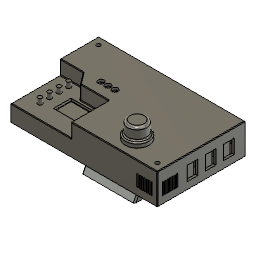
Cover Control Gehäuse (Autodesk Fusion 360 design; units mm, degrees)
Autodesk Fusion 360 part; units mm, degrees
sketch "Skizze1" plane through (0, 0, 0) normal (0, 1, 0) x (1, 0, 0)
  line L0 (0, 0) -> (120, 0)
  line L1 (120, 0) -> (120, -70)
  line L2 (120, -70) -> (0, -70)
  line L3 (0, -70) -> (0, 0)
  circle A0 centre (4, -4) radius 1.6
  circle A1 centre (4, -66) radius 1.6
  circle A2 centre (116, -66) radius 1.6
  circle A3 centre (64, -4) radius 1.6
  dimension "d1" = 120
  dimension "d2" = 70
  dimension "d3" = 3.2
  dimension "d4" = 3.2
  dimension "d5" = 3.2
  dimension "d7" = 3.2
  constraint horizontal L0
  constraint vertical L1
  constraint horizontal L2
  constraint vertical L3
  constraint coincident L0.start L3.end
  measures "d1" distance of L0.start L0.end
  measures "d2" distance of L0.start L2.end
  measures "d3" diameter of A0
  measures "d4" diameter of A1
  measures "d5" diameter of A2
  measures "d7" diameter of A3
extrude "Extrusion1" add sketch "Skizze1" along normal blind 1.6 makes body 1
sketch "Skizze2" plane through (0, 1.6, 0) normal (0, 1, 0) x (-1, 0, 0)
  circle A0 centre (-4, 66) radius 1.6
  circle A1 centre (-64, 4) radius 1.6
  circle A2 centre (-116, 66) radius 1.6
  circle A3 centre (-4, 4) radius 1.6
  line L0 (0, 70) -> (-120, 70)
  line L1 (-120, 70) -> (-120, 0)
  line L2 (-120, 0) -> (0, 0)
  line L3 (0, 0) -> (0, 70)
  line L4 (0, 70) -> (-10, 70)
  line L5 (-10, 70) -> (-10, 60)
  line L6 (-10, 60) -> (0, 60)
  line L7 (0, 60) -> (0, 70)
  line L8 (-10, 60) -> (-10, 51.86)
  line L9 (-10, 51.86) -> (-10, 43.72)
  line L10 (-10, 43.72) -> (-10, 35.58)
  circle A4 centre (-10, 60) radius 1.75
  circle A5 centre (-10, 35.58) radius 1.75
  circle A6 centre (-10, 51.86) radius 1.75
  circle A7 centre (-10, 43.72) radius 1.75
  line L11 (0, 70) -> (-19.44, 70)
  line L12 (-19.44, 70) -> (-19.44, 58)
  line L13 (-19.44, 58) -> (0, 58)
  line L14 (0, 58) -> (0, 70)
  line L15 (-19.44, 58) -> (-46.94, 58)
  line L16 (-46.94, 58) -> (-46.94, 43)
  line L17 (-46.94, 43) -> (-19.44, 43)
  line L18 (-19.44, 43) -> (-19.44, 58)
  line L19 (-120, 70) -> (-94, 70)
  line L20 (-94, 70) -> (-94, 61.2)
  line L21 (-94, 61.2) -> (-120, 61.2)
  line L22 (-120, 61.2) -> (-120, 70)
  circle A8 centre (-94, 61.2) radius 3.5
  line L23 (0, 70) -> (0, 30)
  line L24 (0, 30) -> (-32, 30)
  circle A9 centre (-32, 30) radius 2.4
  line L25 (-32, 30) -> (-38, 30)
  circle A10 centre (-38, 30) radius 2.4
  line L26 (-38, 30) -> (-44, 30)
  circle A11 centre (-44, 30) radius 2.4
  line L27 (0, 0) -> (-16, 0)
  line L28 (-16, 0) -> (-25, 0)
  line L29 (-25, 0) -> (-25, 14)
  line L30 (-25, 14) -> (-16, 14)
  line L31 (-16, 14) -> (-16, 0)
  line L32 (0, 0) -> (-66, 0)
  line L33 (-120, 8) -> (-106, 8)
  line L34 (-106, 8) -> (-106, 17)
  line L35 (-106, 17) -> (-120, 17)
  line L36 (-120, 17) -> (-120, 8)
  line L37 (-120, 17) -> (-120, 23.5)
  line L38 (-120, 23.5) -> (-106, 23.5)
  line L39 (-106, 23.5) -> (-106, 32.5)
  line L40 (-106, 32.5) -> (-120, 32.5)
  line L41 (-120, 32.5) -> (-120, 23.5)
  line L42 (-120, 32.5) -> (-120, 39)
  line L43 (-120, 39) -> (-106, 39)
  line L44 (-106, 39) -> (-106, 48)
  line L45 (-106, 48) -> (-120, 48)
  line L46 (-120, 48) -> (-120, 39)
  line L47 (-120, 70) -> (-118, 70)
  line L48 (-118, 70) -> (-118, 64)
  line L49 (-118, 64) -> (-120, 64)
  line L50 (-120, 64) -> (-120, 70)
  line L51 (-118, 64) -> (-104, 64)
  line L52 (-104, 64) -> (-104, 54)
  line L53 (-104, 54) -> (-118, 54)
  line L54 (-118, 54) -> (-118, 64)
  line L55 (-66, 0) -> (-76, 0)
  line L56 (-76, 0) -> (-76, 10)
  line L57 (-76, 10) -> (-66, 10)
  line L58 (-66, 10) -> (-66, 0)
  line L59 (-120, 0) -> (-76, 0)
  line L60 (-76, 0) -> (-51, 0)
  line L61 (-51, 0) -> (-51, 66)
  line L62 (-51, 66) -> (-76, 66)
  line L63 (-76, 66) -> (-76, 0)
  line L64 (-66, 0) -> (-56, 0)
  line L65 (-56, 0) -> (-56, 10)
  line L66 (-56, 10) -> (-66, 10)
  line L67 (-66, 10) -> (-66, 0)
  dimension "d10" = 10
  dimension "d11" = 10
  dimension "d12" = 8.14
  dimension "d13" = 8.14
  dimension "d14" = 8.14
  dimension "d15" = 3.5
  dimension "d17" = 3.5
  dimension "d18" = 3.5
  dimension "d19" = 3.5
  dimension "d20" = 19.44
  dimension "d21" = 12
  dimension "d22" = 27.5
  dimension "d23" = 15
  dimension "d24" = 26
  dimension "d25" = 8.8
  dimension "d26" = 7
  dimension "d27" = 40
  dimension "d28" = 32
  dimension "d29" = 4.8
  dimension "d30" = 6
  dimension "d31" = 4.8
  dimension "d32" = 6
  dimension "d33" = 4.8
  dimension "d34" = 16
  dimension "d35" = 9
  dimension "d36" = 14
  dimension "d37" = 66
  dimension "d38" = 14
  dimension "d39" = 9
  dimension "d40" = 6.5
  dimension "d41" = 14
  dimension "d42" = 9
  dimension "d43" = 6.5
  dimension "d44" = 14
  dimension "d45" = 9
  dimension "d46" = 2
  dimension "d47" = 6
  dimension "d48" = 14
  dimension "d49" = 10
  dimension "d62" = 10
  dimension "d63" = 10
  dimension "d64" = 44
  dimension "d65" = 25
  dimension "d66" = 66
  dimension "d67" = 10
  dimension "d68" = 10
  constraint horizontal L4
  constraint vertical L5
  constraint horizontal L6
  constraint vertical L7
  constraint coincident L0.start L3.end
  constraint perpendicular L6 L8
  constraint parallel L8 L9
  constraint parallel L9 L10
  constraint coincident L5.end L6.start
  constraint coincident L10.end A5.centre
  constraint coincident L8.end L9.start
  constraint coincident L9.end L10.start
  constraint horizontal L11
  constraint vertical L12
  constraint horizontal L13
  constraint vertical L14
  constraint horizontal L15
  constraint vertical L16
  constraint horizontal L17
  constraint vertical L18
  constraint horizontal L19
  constraint vertical L20
  constraint horizontal L21
  constraint vertical L22
  constraint coincident L0.end L1.start
  constraint coincident L20.end L21.start
  constraint perpendicular L4 L23
  constraint perpendicular L23 L24
  constraint coincident L24.end A9.centre
  constraint parallel L24 L25
  constraint coincident L25.end A10.centre
  constraint parallel L25 L26
  constraint coincident L26.end A11.centre
  constraint coincident L2.end L3.start
  constraint perpendicular L3 L27
  constraint horizontal L28
  constraint vertical L29
  constraint horizontal L30
  constraint vertical L31
  constraint parallel L2 L32
  constraint horizontal L33
  constraint vertical L34
  constraint horizontal L35
  constraint vertical L36
  constraint coincident L1 L33.start
  constraint perpendicular L35 L37
  constraint horizontal L38
  constraint vertical L39
  constraint horizontal L40
  constraint vertical L41
  constraint perpendicular L40 L42
  constraint horizontal L43
  constraint vertical L44
  constraint horizontal L45
  constraint vertical L46
  constraint horizontal L47
  constraint vertical L48
  constraint horizontal L49
  constraint vertical L50
  constraint horizontal L51
  constraint vertical L52
  constraint horizontal L53
  constraint vertical L54
  constraint horizontal L55
  constraint vertical L56
  constraint horizontal L57
  constraint vertical L58
  constraint coincident L1.end L2.start
  constraint perpendicular L1 L59
  constraint horizontal L60
  constraint vertical L61
  constraint horizontal L62
  constraint vertical L63
  constraint horizontal L64
  constraint vertical L65
  constraint horizontal L66
  constraint vertical L67
  measures "d5" diameter of L10.end
  measures "d10" distance of L0.start L4.end
  measures "d11" distance of L0.start L6.end
  measures "d12" distance of L5.end L8.end
  measures "d13" distance of L8.end L9.end
  measures "d14" distance of L9.end L10.end
  measures "d15" diameter of A4
  measures "d17" diameter of A5
  measures "d18" diameter of A6
  measures "d19" diameter of A7
  measures "d20" distance of L0.start L11.end
  measures "d21" distance of L0.start L13.end
  measures "d22" distance of L12.end L15.end
  measures "d23" distance of L12.end L17.end
  measures "d24" distance of L0.end L19.end
  measures "d25" distance of L0.end L21.end
  measures "d26" diameter of A8
  measures "d27" distance of L0.start L23.end
  measures "d28" distance of L23.end L24.end
  measures "d29" diameter of A9
  measures "d30" distance of L24.end L25.end
  measures "d31" diameter of A10
  measures "d32" distance of L25.end L26.end
  measures "d33" diameter of A11
  measures "d34" distance of L2.end L27.end
  measures "d35" distance of L27.end L28.end
  measures "d36" distance of L27.end L30.end
  measures "d37" distance of L2.end L32.end
  measures "d38" distance of L33.start L33.end
  measures "d39" distance of L33.start L35.end
  measures "d40" distance of L35.end L37.end
  measures "d41" distance of L37.end L38.end
  measures "d42" distance of L37.end L40.end
  measures "d43" distance of L40.end L42.end
  measures "d44" distance of L42.end L43.end
  measures "d45" distance of L42.end L45.end
  measures "d46" distance of L0.end L47.end
  measures "d47" distance of L0.end L49.end
  measures "d48" distance of L48.end L51.end
  measures "d49" distance of L48.end L53.end
  measures "d62" distance of L32.end L55.end
  measures "d63" distance of L32.end L57.end
  measures "d64" distance of L1.end L55.end
  measures "d65" distance of L55.end L60.end
  measures "d66" distance of L55.end L62.end
  measures "d67" distance of L32.end L64.end
  measures "d68" distance of L32.end L57.end
  measures "d89" diameter of L35.end
  measures "d93" diameter of L10.end
  measures "d96" diameter of L35.end
extrude "Extrusion2" add sketch "Skizze2" along normal blind 11 contours L2 L28 L29 L30 L31 L32 | L1 L43 L44 L45 L46 | L1 L38 L39 L40 L41 | L1 L33 L34 L35 L36 bodies 1
extrude "Extrusion3" add sketch "Skizze2" along normal blind 5 contours L21 L51 L52 L54 | L21 L52 L53 L54 bodies 1
extrude "Extrusion4" add sketch "Skizze2" along normal blind 6 contours L15 L16 L17 L18 bodies 1
extrude "Extrusion5" add sketch "Skizze2" along normal blind 13 contours L5 L6 A4 | L5 L8 A4 | L6 L8 A4 | L8 L9 A6 | L8 L9 A6 | L9 L10 A7 | L9 L10 A7 | A5 bodies 1
extrude "Extrusion6" add sketch "Skizze2" along normal blind 12.5 contours L24 A9 L25 | L24 A9 L25 | L25 A10 L26 | L25 A10 L26 | A11 bodies 1
extrude "Extrusion7" add sketch "Skizze2" along normal blind 25 contours L20 L21 A8 | L20 L21 A8 bodies 1
extrude "Extrusion8" add sketch "Skizze2" along normal blind 10.3 contours L2 L55 L56 L57 L58 L60 L63 L67 bodies 1
extrude "Extrusion9" add sketch "Skizze2" along normal blind 12.3 contours L2 L32 L58 L60 L64 L65 L66 L67 bodies 1
extrude "Extrusion10" add sketch "Skizze2" along normal blind 9.5 contours L2 L32 L57 L60 L61 L62 L63 L65 L66 bodies 1
sketch "Skizze3" plane through (0, 0, 0) normal (0, 1, 0) x (1, 0, 0)
  line L0 (120, -70) -> (122.5, -70)
  line L1 (122.5, -70) -> (122.5, -72.5)
  line L2 (122.5, -72.5) -> (120, -72.5)
  line L3 (120, -72.5) -> (120, -70)
  line L4 (0, 0) -> (-2.5, 0)
  line L5 (-2.5, 0) -> (-2.5, 2.5)
  line L6 (-2.5, 2.5) -> (0, 2.5)
  line L7 (0, 2.5) -> (0, 0)
  line L8 (-2.5, 2.5) -> (122.5, 2.5)
  line L9 (122.5, 2.5) -> (122.5, -72.5)
  line L10 (122.5, -72.5) -> (-2.5, -72.5)
  line L11 (-2.5, -72.5) -> (-2.5, 2.5)
  dimension "d75" = 2.5
  dimension "d76" = 2.5
  dimension "d77" = 2.5
  dimension "d78" = 2.5
  constraint horizontal L0
  constraint vertical L1
  constraint horizontal L2
  constraint vertical L3
  constraint horizontal L4
  constraint vertical L5
  constraint horizontal L6
  constraint vertical L7
  constraint coincident L4.start L7.end
  constraint horizontal L8
  constraint vertical L9
  constraint horizontal L10
  constraint vertical L11
  measures "d75" distance of L0.start L0.end
  measures "d76" distance of L0.start L2.end
  measures "d77" distance of L4.start L4.end
  measures "d78" distance of L4.start L6.end
extrude "Extrusion11" add sketch "Skizze3" along normal blind 22 separate body makes body 2
sketch "Skizze4" plane through (0, 22, 0) normal (0, 1, 0) x (-1, 0, 0)
  line L0 (2.5, 72.5) -> (-122.5, 72.5)
  line L1 (-122.5, 72.5) -> (-122.5, -2.5)
  line L2 (-122.5, -2.5) -> (2.5, -2.5)
  line L3 (2.5, -2.5) -> (2.5, 72.5)
  line L4 (2.5, 72.5) -> (-49, 72.5)
  line L5 (-49, 72.5) -> (-49, 40.5)
  line L6 (-49, 40.5) -> (-25, 40.5)
  line L7 (-25, 40.5) -> (-17.4344, 30.5702)
  line L8 (-17.4344, 30.5702) -> (2.5, 30.5702)
  dimension "d81" = 51.5
  dimension "d82" = 32
  dimension "d83" = 24
  constraint coincident L0.start L3.end
  constraint perpendicular L3 L4
  constraint perpendicular L4 L5
  constraint perpendicular L5 L6
  constraint coincident L3 L8.end
  constraint perpendicular L3 L8
  measures "d81" distance of L0.start L4.end
  measures "d82" distance of L4.end L5.end
  measures "d83" distance of L5.end L6.end
extrude "Extrusion12" cut sketch "Skizze4" against normal blind 12 contours L0 L3 L4 L5 L6 L7 L8 bodies 2
shell "Schale1" thickness 2 removed faces 1 at (80.8333, 0, 47.5) on bodies 2
sketch "Skizze6" plane through (0, 20, 0) normal (0, -1, 0) x (1, 0, 0)
  line L0 (51, 70.5) -> (51, 38.5)
  line L1 (51, 38.5) -> (25.9905, 38.5)
  line L2 (25.9905, 38.5) -> (18.425, 28.5702)
  line L3 (18.425, 28.5702) -> (-0.5, 28.5702)
  line L4 (-0.5, 28.5702) -> (-0.5, -0.5)
  line L5 (-0.5, -0.5) -> (120.5, -0.5)
  line L6 (120.5, -0.5) -> (120.5, 70.5)
  line L7 (120.5, 70.5) -> (51, 70.5)
  line L8 (120.5, 70.5) -> (102.5114, 70.5)
  line L9 (102.5114, 70.5) -> (102.5114, 51.9822)
  line L10 (102.5114, 51.9822) -> (120.5, 51.9822)
  line L11 (120.5, 51.9822) -> (120.5, 70.5)
  line L12 (120.5, 70.5) -> (101.404, 70.5)
  line L13 (101.404, 70.5) -> (101.404, 51.0001)
  line L14 (101.404, 51.0001) -> (120.5, 51.0001)
  line L15 (120.5, 51.0001) -> (120.5, 70.5)
  constraint horizontal L8
  constraint vertical L9
  constraint horizontal L10
  constraint vertical L11
  constraint coincident L6.end L7.start
  constraint horizontal L12
  constraint vertical L13
  constraint horizontal L14
  constraint vertical L15
extrude "Extrusion13" add sketch "Skizze6" along normal blind 18 contours L6 L7 L9 L10 L12 L13 L14 L15 bodies 2
sketch "Skizze7" plane through (0, 10, 0) normal (0, 1, 0) x (-1, 0, 0)
  line L0 (-17.4344, 30.5702) -> (2.5, 30.5702)
  line L1 (2.5, 30.5702) -> (2.5, 72.5)
  line L2 (2.5, 72.5) -> (-49, 72.5)
  line L3 (-49, 72.5) -> (-49, 40.5)
  line L4 (-49, 40.5) -> (-25, 40.5)
  line L5 (-25, 40.5) -> (-17.4344, 30.5702)
  line L6 (-19.5, 42.9671) -> (-47, 42.9671)
  line L7 (-47, 42.9671) -> (-47, 57.9671)
  line L8 (-47, 57.9671) -> (-19.5, 57.9671)
  line L9 (-19.5, 57.9671) -> (-19.5, 42.9671)
  circle A0 centre (-10, 60) radius 1.9
  circle A1 centre (-10, 35.6) radius 1.9
  circle A2 centre (-9.9957, 43.7481) radius 1.9
  circle A3 centre (-10, 51.85) radius 1.9
  dimension "d89" = 3.8
  dimension "d91" = 3.8
  dimension "d92" = 3.8
  dimension "d93" = 3.8
  constraint horizontal L6
  constraint vertical L7
  constraint horizontal L8
  constraint vertical L9
  measures "d89" diameter of A0
  measures "d91" diameter of A1
  measures "d92" diameter of A2
  measures "d93" diameter of A3
extrude "Extrusion14" cut sketch "Skizze7" against normal blind 2 contours L6 L7 L8 L9 | A0 | A1 | A2 | A3 bodies 2
sketch "Skizze8" plane through (0, 22, 0) normal (0, 1, 0) x (-1, 0, 0)
  line L0 (-49, 40.5) -> (-49, 72.5)
  line L1 (-49, 72.5) -> (-122.5, 72.5)
  line L2 (-122.5, 72.5) -> (-122.5, -2.5)
  line L3 (-122.5, -2.5) -> (2.5, -2.5)
  line L4 (2.5, -2.5) -> (2.5, 30.5702)
  line L5 (2.5, 30.5702) -> (-17.4344, 30.5702)
  line L6 (-17.4344, 30.5702) -> (-25, 40.5)
  line L7 (-25, 40.5) -> (-49, 40.5)
  circle A0 centre (-44, 30) radius 2.5
  circle A1 centre (-38, 30) radius 2.5
  circle A2 centre (-32, 30) radius 2.5
  circle A3 centre (-94.0122, 61.2049) radius 3.6
  circle A4 centre (-4, 4) radius 1.6
  circle A5 centre (-116.0155, 65.9809) radius 1.6
  circle A6 centre (-116.0155, 65.9809) radius 3.5
  circle A7 centre (-4, 4) radius 3.5
  line L8 (-112.8531, 64.4812) -> (-119.1779, 64.4812)
  dimension "d96" = 5
  dimension "d97" = 5
  dimension "d98" = 5
  dimension "d99" = 7.2
  dimension "d176" = 3.2
  dimension "d177" = 3.2
  dimension "d214" = 7
  dimension "d215" = 7
  constraint concentric A5 A6
  constraint concentric A4 A7
  constraint coincident A6 L8.start
  constraint coincident A6 L8.end
  constraint horizontal L8
  measures "d96" diameter of A0
  measures "d97" diameter of A1
  measures "d98" diameter of A2
  measures "d99" diameter of A3
  measures "d176" diameter of A4
  measures "d177" diameter of A5
  measures "d214" diameter of A6
  measures "d215" diameter of A7
extrude "Extrusion15" cut sketch "Skizze8" against normal blind 2 contours A0 | A1 | A2 | A3 bodies 2
sketch "Skizze9" plane through (122.5, 0, 0) normal (1, 0, 0) x (0, 0, -1)
  line L0 (-72.5, 0) -> (2.5, 0)
  line L1 (2.5, 0) -> (2.5, 22)
  line L2 (2.5, 22) -> (-72.5, 22)
  line L3 (-72.5, 22) -> (-72.5, 0)
  line L4 (-7, 2) -> (-16, 2)
  line L5 (-16, 2) -> (-16, 14)
  line L6 (-16, 14) -> (-7, 14)
  line L7 (-7, 14) -> (-7, 2)
  line L8 (-22.5, 2) -> (-31.5, 2)
  line L9 (-31.5, 2) -> (-31.5, 14)
  line L10 (-31.5, 14) -> (-22.5, 14)
  line L11 (-22.5, 14) -> (-22.5, 2)
  line L12 (-38, 2) -> (-47, 2)
  line L13 (-47, 2) -> (-47, 14)
  line L14 (-47, 14) -> (-38, 14)
  line L15 (-38, 14) -> (-38, 2)
  line L16 (-55.0817, 2.0257) -> (-56.0817, 2.0257)
  line L17 (-56.0817, 2.0257) -> (-56.0817, 12.0257)
  line L18 (-56.0817, 12.0257) -> (-55.0817, 12.0257)
  line L19 (-55.0817, 12.0257) -> (-55.0817, 2.0257)
  line L20 (-57.0817, 2.0257) -> (-58.0817, 2.0257)
  line L21 (-58.0817, 2.0257) -> (-58.0817, 12.0257)
  line L22 (-58.0817, 12.0257) -> (-57.0817, 12.0257)
  line L23 (-57.0817, 12.0257) -> (-57.0817, 2.0257)
  line L24 (-59.0817, 2.0257) -> (-60.0817, 2.0257)
  line L25 (-60.0817, 2.0257) -> (-60.0817, 12.0257)
  line L26 (-60.0817, 12.0257) -> (-59.0817, 12.0257)
  line L27 (-59.0817, 12.0257) -> (-59.0817, 2.0257)
  line L28 (-61.0817, 2.0257) -> (-62.0817, 2.0257)
  line L29 (-62.0817, 2.0257) -> (-62.0817, 12.0257)
  line L30 (-62.0817, 12.0257) -> (-61.0817, 12.0257)
  line L31 (-61.0817, 12.0257) -> (-61.0817, 2.0257)
  line L32 (-63.0817, 2.0257) -> (-64.0817, 2.0257)
  line L33 (-64.0817, 2.0257) -> (-64.0817, 12.0257)
  line L34 (-64.0817, 12.0257) -> (-63.0817, 12.0257)
  line L35 (-63.0817, 12.0257) -> (-63.0817, 2.0257)
  line L36 (-65.0817, 2.0257) -> (-66.0817, 2.0257)
  line L37 (-66.0817, 2.0257) -> (-66.0817, 12.0257)
  line L38 (-66.0817, 12.0257) -> (-65.0817, 12.0257)
  line L39 (-65.0817, 12.0257) -> (-65.0817, 2.0257)
  line L40 (-67.0817, 2.0257) -> (-68.0817, 2.0257)
  line L41 (-68.0817, 2.0257) -> (-68.0817, 12.0257)
  line L42 (-68.0817, 12.0257) -> (-67.0817, 12.0257)
  line L43 (-67.0817, 12.0257) -> (-67.0817, 2.0257)
  line L44 (2.5, 0) -> (-7, 0)
  line L45 (-7, 0) -> (-7, 2)
  line L46 (-7, 2) -> (2.5, 2)
  line L47 (2.5, 2) -> (2.5, 0)
  line L48 (-16, 2) -> (-22.5, 2)
  line L49 (-31.5, 2) -> (-38, 2)
  dimension "d102" = 9
  dimension "d103" = 12
  dimension "d104" = 9
  dimension "d105" = 12
  dimension "d106" = 9
  dimension "d107" = 12
  dimension "d108" = 1
  dimension "d109" = 10
  dimension "d110" = 1
  dimension "d111" = 10
  dimension "d112" = 10
  dimension "d113" = 1
  dimension "d114" = 10
  dimension "d115" = 1
  dimension "d116" = 10
  dimension "d117" = 1
  dimension "d118" = 10
  dimension "d119" = 1
  dimension "d120" = 10
  dimension "d218" = 9.5
  dimension "d219" = 2
  dimension "d220" = 6.5
  dimension "d221" = 6.5
  constraint horizontal L4
  constraint vertical L5
  constraint horizontal L6
  constraint vertical L7
  constraint horizontal L8
  constraint vertical L9
  constraint horizontal L10
  constraint vertical L11
  constraint horizontal L12
  constraint vertical L13
  constraint horizontal L14
  constraint vertical L15
  constraint horizontal L16
  constraint vertical L17
  constraint horizontal L18
  constraint vertical L19
  constraint horizontal L20
  constraint vertical L21
  constraint horizontal L22
  constraint vertical L23
  constraint horizontal L24
  constraint vertical L25
  constraint horizontal L26
  constraint vertical L27
  constraint horizontal L28
  constraint vertical L29
  constraint horizontal L30
  constraint vertical L31
  constraint horizontal L32
  constraint vertical L33
  constraint horizontal L34
  constraint vertical L35
  constraint horizontal L36
  constraint vertical L37
  constraint horizontal L38
  constraint vertical L39
  constraint horizontal L40
  constraint vertical L41
  constraint horizontal L42
  constraint vertical L43
  constraint horizontal L44
  constraint vertical L45
  constraint horizontal L46
  constraint vertical L47
  constraint coincident L0.end L1.start
  constraint coincident L4.start L7.end
  constraint perpendicular L5 L48
  constraint coincident L8.start L11.end
  constraint perpendicular L9 L49
  constraint coincident L12.start L15.end
  measures "d102" distance of L4.start L4.end
  measures "d103" distance of L4.start L6.end
  measures "d104" distance of L8.start L8.end
  measures "d105" distance of L8.start L10.end
  measures "d106" distance of L12.start L12.end
  measures "d107" distance of L12.start L14.end
  measures "d108" distance of L16.start L16.end
  measures "d109" distance of L16.start L18.end
  measures "d110" distance of L20.start L20.end
  measures "d111" distance of L20.start L22.end
  measures "d112" distance of L24.start L26.end
  measures "d113" distance of L28.start L28.end
  measures "d114" distance of L28.start L30.end
  measures "d115" distance of L32.start L32.end
  measures "d116" distance of L32.start L34.end
  measures "d117" distance of L36.start L36.end
  measures "d118" distance of L36.start L38.end
  measures "d119" distance of L40.start L40.end
  measures "d120" distance of L40.start L42.end
  measures "d218" distance of L0.end L44.end
  measures "d219" distance of L0.end L46.end
  measures "d220" distance of L4.end L8.start
  measures "d221" distance of L8.end L12.start
extrude "Extrusion16" cut sketch "Skizze9" against normal blind 2 contours L4 L5 L6 L7 | L8 L9 L10 L11 | L12 L13 L14 L15 | L16 L17 L18 L19 | L20 L21 L22 L23 | L24 L25 L26 L27 | L28 L29 L30 L31 | L32 L33 L34 L35 | L36 L37 L38 L39 | L40 L41 L42 L43 bodies 2
sketch "Skizze10" plane through (0, 0, -2.5) normal (0, 0, -1) x (-1, 0, 0)
  line L0 (-122.5, 0) -> (2.5, 0)
  line L1 (2.5, 0) -> (2.5, 22)
  line L2 (2.5, 22) -> (-122.5, 22)
  line L3 (-122.5, 22) -> (-122.5, 0)
  line L4 (-78, 14.5) -> (-64, 14.5)
  line L5 (-64, 14.5) -> (-64, 6.5)
  line L6 (-64, 6.5) -> (-78, 6.5)
  line L7 (-78, 6.5) -> (-78, 14.5)
  line L8 (-15, 2) -> (-24, 2)
  line L9 (-24, 2) -> (-24, 14)
  line L10 (-24, 14) -> (-15, 14)
  line L11 (-15, 14) -> (-15, 2)
  line L12 (2.5, 0) -> (-15, 0)
  line L13 (-15, 0) -> (-15, 2)
  line L14 (-15, 2) -> (2.5, 2)
  line L15 (2.5, 2) -> (2.5, 0)
  line L16 (-24, 2) -> (-64, 2)
  line L17 (-64, 2) -> (-64, 6.5)
  line L18 (-64, 6.5) -> (-24, 6.5)
  line L19 (-24, 6.5) -> (-24, 2)
  dimension "d123" = 14
  dimension "d124" = 8
  dimension "d125" = 9
  dimension "d126" = 12
  dimension "d222" = 17.5
  dimension "d223" = 2
  dimension "d224" = 40
  dimension "d225" = 4.5
  constraint horizontal L4
  constraint vertical L5
  constraint horizontal L6
  constraint vertical L7
  constraint horizontal L8
  constraint vertical L9
  constraint horizontal L10
  constraint vertical L11
  constraint horizontal L12
  constraint vertical L13
  constraint horizontal L14
  constraint vertical L15
  constraint coincident L0.end L1.start
  constraint coincident L8.start L11.end
  constraint horizontal L16
  constraint vertical L17
  constraint horizontal L18
  constraint vertical L19
  constraint coincident L5.end L6.start
  measures "d123" distance of L4.start L4.end
  measures "d124" distance of L4.start L6.end
  measures "d125" distance of L8.start L8.end
  measures "d126" distance of L8.start L10.end
  measures "d222" distance of L0.end L12.end
  measures "d223" distance of L0.end L14.end
  measures "d224" distance of L8.end L16.end
  measures "d225" distance of L8.end L18.end
extrude "Extrusion17" cut sketch "Skizze10" against normal blind 2 contours L4 L5 L6 L7 | L8 L9 L10 L11 L19 bodies 2
fillet "Abrundung1" radius 2 1 edges at (78, 14.5, -1.5) on bodies 2
fillet "Abrundung2" radius 2 1 edges at (78, 6.5, -1.5) on bodies 2
fillet "Abrundung3" radius 2 1 edges at (64, 6.5, -1.5) on bodies 2
fillet "Abrundung4" radius 2 1 edges at (64, 14.5, -1.5) on bodies 2
sketch "Skizze11" plane through (0, 0, 72.5) normal (0, 0, 1) x (1, 0, 0)
  line L0 (49, 22) -> (49, 10)
  line L1 (49, 10) -> (-2.5, 10)
  line L2 (-2.5, 10) -> (-2.5, 0)
  line L3 (-2.5, 0) -> (122.5, 0)
  line L4 (122.5, 0) -> (122.5, 22)
  line L5 (122.5, 22) -> (49, 22)
  line L6 (118, 2) -> (117, 2)
  line L7 (117, 2) -> (117, 12)
  line L8 (117, 12) -> (118, 12)
  line L9 (118, 12) -> (118, 2)
  line L10 (116, 2) -> (115, 2)
  line L11 (115, 2) -> (115, 12)
  line L12 (115, 12) -> (116, 12)
  line L13 (116, 12) -> (116, 2)
  line L14 (114, 2) -> (113, 2)
  line L15 (113, 2) -> (113, 12)
  line L16 (113, 12) -> (114, 12)
  line L17 (114, 12) -> (114, 2)
  line L18 (112, 2) -> (111, 2)
  line L19 (111, 2) -> (111, 12)
  line L20 (111, 12) -> (112, 12)
  line L21 (112, 12) -> (112, 2)
  line L22 (110, 2) -> (109, 2)
  line L23 (109, 2) -> (109, 12)
  line L24 (109, 12) -> (110, 12)
  line L25 (110, 12) -> (110, 2)
  line L26 (108, 2) -> (107, 2)
  line L27 (107, 2) -> (107, 12)
  line L28 (107, 12) -> (108, 12)
  line L29 (108, 12) -> (108, 2)
  line L30 (106, 2) -> (105, 2)
  line L31 (105, 2) -> (105, 12)
  line L32 (105, 12) -> (106, 12)
  line L33 (106, 12) -> (106, 2)
  dimension "d137" = 1
  dimension "d138" = 10
  dimension "d139" = 1
  dimension "d140" = 10
  dimension "d141" = 1
  dimension "d142" = 10
  dimension "d143" = 1
  dimension "d144" = 10
  dimension "d145" = 1
  dimension "d146" = 10
  dimension "d147" = 1
  dimension "d148" = 10
  dimension "d149" = 1
  dimension "d150" = 10
  constraint horizontal L6
  constraint vertical L7
  constraint horizontal L8
  constraint vertical L9
  constraint horizontal L10
  constraint vertical L11
  constraint horizontal L12
  constraint vertical L13
  constraint horizontal L14
  constraint vertical L15
  constraint horizontal L16
  constraint vertical L17
  constraint horizontal L18
  constraint vertical L19
  constraint horizontal L20
  constraint vertical L21
  constraint horizontal L22
  constraint vertical L23
  constraint horizontal L24
  constraint vertical L25
  constraint horizontal L26
  constraint vertical L27
  constraint horizontal L28
  constraint vertical L29
  constraint horizontal L30
  constraint vertical L31
  constraint horizontal L32
  constraint vertical L33
  measures "d137" distance of L6.start L6.end
  measures "d138" distance of L6.start L8.end
  measures "d139" distance of L10.start L10.end
  measures "d140" distance of L10.start L12.end
  measures "d141" distance of L14.start L14.end
  measures "d142" distance of L14.start L16.end
  measures "d143" distance of L18.start L18.end
  measures "d144" distance of L18.start L20.end
  measures "d145" distance of L22.start L22.end
  measures "d146" distance of L22.start L24.end
  measures "d147" distance of L26.start L26.end
  measures "d148" distance of L26.start L28.end
  measures "d149" distance of L30.start L30.end
  measures "d150" distance of L30.start L32.end
extrude "Extrusion18" cut sketch "Skizze11" against normal blind 2 contours L6 L7 L8 L9 | L10 L11 L12 L13 | L14 L15 L16 L17 | L18 L19 L20 L21 | L22 L23 L24 L25 | L26 L27 L28 L29 | L30 L31 L32 L33 bodies 2
extrude "Extrusion19" add 1 faces at (80.1667, 0, 71.8333) along direction (0, -1, 0) blind 2 on bodies 2 bodies 2
sketch "Skizze12" plane through (0, -2, 0) normal (0, -1, 0) x (1, 0, 0)
  line L0 (-0.5, 70.5) -> (120.5, 70.5)
  line L1 (120.5, 70.5) -> (120.5, -0.5)
  line L2 (120.5, -0.5) -> (-0.5, -0.5)
  line L3 (-0.5, -0.5) -> (-0.5, 70.5)
  line L4 (122.5, 72.5) -> (-2.5, 72.5)
  line L5 (-2.5, 72.5) -> (-2.5, -2.5)
  line L6 (-2.5, -2.5) -> (122.5, -2.5)
  line L7 (122.5, -2.5) -> (122.5, 72.5)
  line L8 (-2.5, -2.5) -> (122.5, -2.5)
  line L9 (122.5, -2.5) -> (122.5, 72.5)
  line L10 (122.5, 72.5) -> (-2.5, 72.5)
  line L11 (-2.5, 72.5) -> (-2.5, -2.5)
  circle A0 centre (64, 4) radius 3
  circle A1 centre (4, 4) radius 3.5
  circle A2 centre (3.9884, 65.9924) radius 3
  circle A3 centre (116, 66) radius 3.5
  circle A4 centre (64, 4) radius 1.5
  circle A5 centre (3.9884, 65.9924) radius 1.5
  circle A6 centre (116, 66) radius 2.1
  circle A7 centre (4, 4) radius 2.1
  line L12 (-2.5, 72.5) -> (122.5, -2.5)
  line L13 (122.5, 72.5) -> (-2.5, -2.5)
  line L14 (60, 35) -> (50, 35)
  line L15 (60, 35) -> (70, 35)
  circle A8 centre (50, 35) radius 1.6
  circle A9 centre (70, 35) radius 1.6
  circle A10 centre (50, 35) radius 2.1
  circle A11 centre (70, 35) radius 2.1
  circle A12 centre (50, 35) radius 1.5
  circle A13 centre (70, 35) radius 1.5
  dimension "d157" = 6
  dimension "d158" = 7
  dimension "d159" = 6
  dimension "d160" = 7
  dimension "d163" = 3
  dimension "d164" = 3
  dimension "d169" = 4.2
  dimension "d170" = 4.2
  dimension "d194" = 10
  dimension "d195" = 10
  dimension "d196" = 3.2
  dimension "d197" = 3.2
  dimension "d209" = 4.2
  dimension "d210" = 4.2
  dimension "d247" = 3
  dimension "d248" = 3
  constraint horizontal L8
  constraint vertical L9
  constraint horizontal L10
  constraint vertical L11
  constraint coincident L4.start L7.end
  constraint coincident L5.end L6.start
  constraint concentric A0 A4
  constraint concentric A2 A5
  constraint concentric A3 A6
  constraint concentric A1 A7
  constraint coincident L4.end L5.start
  constraint coincident L6.end L7.start
  constraint midpoint L13 L14.start
  constraint perpendicular L3 L14
  constraint parallel L14 L15
  constraint coincident L14.end A8.centre
  constraint coincident L15.end A9.centre
  constraint concentric A8 A10
  constraint concentric A9 A11
  constraint concentric A8 A12
  constraint concentric A11 A13
  measures "d157" diameter of A0
  measures "d158" diameter of A1
  measures "d159" diameter of A2
  measures "d160" diameter of A3
  measures "d163" diameter of A4
  measures "d164" diameter of A5
  measures "d169" diameter of A6
  measures "d170" diameter of A7
  measures "d194" distance of L14.start L14.end
  measures "d195" distance of L14.start L15.end
  measures "d196" diameter of A8
  measures "d197" diameter of A9
  measures "d209" diameter of A10
  measures "d210" diameter of A11
  measures "d247" diameter of A12
  measures "d248" diameter of A13
extrude "Extrusion20" add sketch "Skizze12" along normal blind 2 separate body contours L0 L2 L3 L5 L11 L12 L13 | L0 L2 L3 A1 A2 L12 L13 | L0 L4 L10 L12 L13 | L0 A2 A3 L12 L13 | L0 L1 L2 L7 L9 L12 L13 | L0 L1 L2 A3 L12 L13 | A2 L12 | A2 L12 | L2 A1 L12 L13 | L2 L6 L8 L12 L13 | A3 L13 | A3 L13 | A1 L13 | A1 L13 | A0 | A4 | A5 | A6 | A7 | A8 | A9 | A10 | A11 | A12 | A13 makes body 3
extrude "Extrusion21" add sketch "Skizze12" against normal blind 2 contours A2 L12 | A2 L12 | A3 L13 | A3 L13 | A1 L13 | A1 L13 | A0 | A4 | A5 | A6 | A7 bodies 3
extrude "Extrusion22" add sketch "Skizze12" against normal blind 5 contours A4 | A5 bodies 3
chamfer "Fase1" distance 0.5 angle 45 1 edges at (62.6015, 3, 4.5424) on bodies 3
chamfer "Fase2" distance 0.5 angle 45 1 edges at (2.5899, 3, 66.5348) on bodies 3
extrude "Extrusion23" cut sketch "Skizze12" along normal blind 5 and the other way blind 5 contours A6 | A7 bodies 3
chamfer "Fase3" distance 2 angle 45 4 edges at (60, -2, -2.5) (122.5, -2, 35) (60, -2, 72.5) (-2.5, -2, 35) on bodies 3
extrude "Extrusion24" cut sketch "Skizze8" against normal blind 2 contours A4 | A5 L8 | A5 L8 bodies 2
fillet "Abrundung5" radius 0.5 5 edges at (-2.5, 16, 30.5702) (17.4344, 16, 30.5702) (25, 16, 40.5) (49, 16, 40.5) (49, 16, 72.5) on bodies 2
fillet "Abrundung6" radius 0.5 2 edges at (23.5, 10, 72.5) (-2.5, 10, 51.2851) on bodies 2
fillet "Abrundung7" radius 0.5 11 edges at (-2.5, 22, 13.7851) (-2.3536, 22, 30.4237) (7.5934, 22, 30.5702) (17.4087, 22, 30.6221) (21.2172, 22, 35.5351) (25.0257, 22, 40.4481) (36.8738, 22, 40.5) (48.8536, 22, 40.6464) (49, 22, 56.5) (49.1464, 22, 72.3536) (86, 22, 72.5) on bodies 2
fillet "Abrundung8" radius 0.5 9 edges at (-2.3536, 9.8536, 30.4237) (7.5934, 10, 30.5702) (17.4087, 10, 30.6221) (21.2172, 10, 35.5351) (25.0257, 10, 40.4481) (36.8738, 10, 40.5) (48.8536, 10, 40.6464) (49, 10, 56.5) (49.1464, 9.8536, 72.3536) on bodies 2
fillet "Abrundung9" radius 0.5 6 edges at (60.25, 22, -2.5) (-2.3536, 21.8536, -2.5) (-2.5, 9.75, -2.5) (122.5, 9.75, 72.5) (122.5, 21.8536, 72.3536) (122.5, 22, 34.75) on bodies 2
extrude "Extrusion25" add 1 faces at (39.6667, -2, 71.8333) along direction (0, -1, 0) blind 2 on bodies 2 bodies 2
chamfer "Fase4" distance 2 angle 45 4 edges at (60, -4, 70.5) (-0.5, -4, 35) (60, -4, -0.5) (120.5, -4, 35) on bodies 2
ref_plane "Arbeitsebene1" through (62.5, 8.75, 34.75) normal (1, 0, 0) x (0, 0, -1)
extrude "Extrusion26" cut sketch "Skizze12" along normal blind 2 contours A8 | A9 | A12 | A13 bodies 3
sketch "Skizze13" plane through (62.5, 0, 0) normal (1, 0, 0) x (0, 0, -1)
  line L0 (-35, -2) -> (-23, -2)
  line L1 (-23, -2) -> (-23, -4)
  line L2 (-23, -4) -> (-47, -4)
  line L3 (-47, -4) -> (-47, -22)
  line L4 (-47, -22) -> (-23, -22)
  line L5 (-23, -22) -> (-23, -4)
  line L6 (-47, -22) -> (-23, -22)
  line L7 (-23, -22) -> (-23, -32)
  line L8 (-23, -32) -> (-47, -32)
  line L9 (-47, -32) -> (-47, -22)
  line L10 (-23, -32) -> (-18, -32)
  line L11 (-18, -32) -> (-23, -22)
  line L12 (-47, -32) -> (-52, -32)
  line L13 (-52, -32) -> (-47, -22)
  dimension "d200" = 12
  dimension "d201" = 24
  dimension "d202" = 18
  dimension "d203" = 24
  dimension "d204" = 10
  dimension "d205" = 5
  dimension "d206" = 5
  constraint horizontal L0
  constraint perpendicular L0 L1
  constraint horizontal L2
  constraint vertical L3
  constraint horizontal L4
  constraint vertical L5
  constraint horizontal L6
  constraint vertical L7
  constraint horizontal L8
  constraint vertical L9
  constraint perpendicular L7 L10
  constraint perpendicular L9 L12
  measures "d200" distance of L0.start L0.end
  measures "d201" distance of L1.end L2.end
  measures "d202" distance of L1.end L4.end
  measures "d203" distance of L3.end L4.end
  measures "d204" distance of L3.end L8.end
  measures "d205" distance of L7.end L10.end
  measures "d206" distance of L8.end L12.end
extrude "Extrusion27" add sketch "Skizze13" along normal blind 20 and the other way blind 25 separate body makes body 4
extrude "Extrusion28" add sketch "Skizze12" along normal blind 10 contours A12 | A13 bodies 4
chamfer "Fase5" distance 1 angle 45 8 edges at (82.5, -13, 23) (82.5, -27, 20.5) (82.5, -27, 49.5) (82.5, -13, 47) (37.5, -13, 47) (37.5, -27, 49.5) (37.5, -27, 20.5) (37.5, -13, 23) on bodies 4
extrude "Extrusion29" add sketch "Skizze8" against normal blind 20.4 contours A5 A6 L8 | A7 picked at (-118.4863, 67.4216) bodies 2
sketch "Skizze14" plane through (0, 26.6, 0) normal (0, 1, 0) x (-1, 0, 0)
  circle A0 centre (-94, 61.2) radius 3.5
  circle A1 centre (-94, 61.2) radius 3
  line L0 (-97, 61.2) -> (-92.4, 61.2)
  circle A2 centre (-94, 61.2) radius 4
  line L1 (-92.4, 57.5339) -> (-92.4, 64.8661)
  line L2 (-94, 61.2) -> (-94, 60.7)
  line L3 (-94, 60.7) -> (-98, 60.7)
  line L4 (-98, 60.7) -> (-98, 61.7)
  line L5 (-98, 61.7) -> (-94, 61.7)
  line L6 (-94, 61.7) -> (-94, 60.7)
  circle A3 centre (-94, 61.2) radius 5
  circle A4 centre (-94, 61.2) radius 10
  dimension "d228" = 6
  dimension "d229" = 4.6
  dimension "d230" = 8
  dimension "d231" = 0.5
  dimension "d232" = 4
  dimension "d233" = 1
  dimension "d234" = 10
  dimension "d235" = 20
  constraint concentric A0 A1
  constraint coincident A1 L0.start
  constraint coincident A0.centre L0
  constraint concentric A1 A2
  constraint coincident A2 L1.start
  constraint coincident A2 L1.end
  constraint vertical L1
  constraint horizontal L0
  constraint coincident L0.end L1
  constraint coincident A0.centre A1.centre
  constraint perpendicular L0 L2
  constraint horizontal L3
  constraint vertical L4
  constraint horizontal L5
  constraint vertical L6
  constraint concentric A1 A3
  constraint concentric A2 A4
  measures "d228" diameter of A1
  measures "d229" distance of L0.start L0.end
  measures "d230" diameter of A2
  measures "d231" distance of A0.centre L2.end
  measures "d232" distance of L2.end L3.end
  measures "d233" distance of L2.end L5.end
  measures "d234" diameter of A3
  measures "d235" diameter of A4
extrude "Extrusion30" add sketch "Skizze14" along normal blind 4 separate body contours A0 A1 L1 | A0 A2 L1 | A0 A1 L1 L5 | A0 A2 L1 L5 | A0 A2 L1 L3 | A0 A1 L1 L3 | A1 L1 | A4 makes body 5 at (84.0497, 27.9333, 60.2043) makes body 6 at (97.9006, 29.2667, 60.3137)
sketch "Skizze15" plane through (0, 30.6, 0) normal (0, 1, 0) x (-1, 0, 0)
  circle A0 centre (-94, 61.2) radius 5
  circle A1 centre (-94, 61.2) radius 10
  circle A2 centre (-94, 61.2) radius 8
  dimension "d238" = 16
  constraint concentric A0 A2
  measures "d238" diameter of A2
extrude "Extrusion31" add sketch "Skizze15" along normal blind 10 contours A0 | A2 bodies 5 6
fillet "Abrundung10" radius 2 1 edges at (101.4586, 40.6, 58.3071) on bodies 5
fillet "Abrundung11" radius 1 1 edges at (101.4586, 30.6, 64.0929) on bodies 5
fillet "Abrundung12" radius 1 1 edges at (103.3233, 30.6, 57.5838) on bodies 5
named bodies: "Cover Control", "Gehäuse Oben", "Gehäuse Unten", "Haltefuß", "Knopf"
